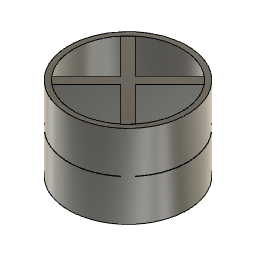
Moen Faucet Tool v1 (Autodesk Fusion 360 design; units mm, degrees)
Autodesk Fusion 360 part; units mm, degrees
note: some values were not read from the file. Set by a fixed rule: which sketch regions a step uses.
sketch "Tool" plane through (0, 0, 0) normal (0, 0, 1) x (1, 0, 0)
  circle A0 centre (0, 0) radius 10.415
  circle A1 centre (0, 0) radius 9.6
  line L0 (-10.415, 0.0013) -> (10.415, 0.0013) construction
  line L1 (0, 10.485) -> (0, -10.415) construction
  line L2 (-10.415, -0.7737) -> (10.415, -0.7737)
  line L3 (-10.415, 0.7763) -> (10.415, 0.7763)
  line L4 (-0.775, 10.485) -> (-0.775, -10.415)
  line L5 (0.775, 10.485) -> (0.775, -10.415)
  circle A2 centre (0, 0) radius 11.415
  dimension "d5" = 20.83
  dimension "d6" = 19.2
  dimension "d7" = 0.775
  dimension "d8" = -0.775
  dimension "d9" = 0.775
  dimension "d10" = -0.775
  dimension "d13" = 1
  constraint coincident A0.centre A1.centre
  constraint concentric A0 A1
  constraint coincident A0 L0.end
  constraint horizontal L0
  constraint coincident A0 L0.start
  constraint coincident A0 L1.end
  constraint perpendicular L0 L1
  measures "d5" diameter of A0
  measures "d6" diameter of A1
extrude "Extrude1" add sketch "Tool" against normal blind 8 contours A0 A1 L2 L3 | A0 A1 L4 L5 | A0 A1 L4 L5 | A0 A1 L2 L3 | A2
move_face "OffsetFaces1" offset -0.05 17 faces at (10.7291, 0.0008, 0) (1.7545, 10.2662, -5.3333) (9.5752, 0.6902, -5.3333) (8.0289, -6.6339, -5.3333) (9.8411, 0.7763, -2.6667) (9.8413, -0.7737, -2.6667) (0.775, 10.1136, -5.3333) (-0.603, 9.581, -5.3333) (-7.0069, 7.7056, -5.3333) (-10.1137, -0.7737, -2.6667) (-0.775, 10.1136, -2.6667) (0.775, -9.8412, -5.3333) (0.603, -9.581, -5.3333) (-1.2662, -10.3377, -5.3333) (-9.5904, -0.4296, -5.3333) (-0.775, -9.8412, -2.6667) (-10.1135, 0.7763, -2.6667)
sketch "Sketch2" plane through (0, 0, -0.05) normal (0, 0, 1) x (-1, 0, 0)
  arc A0 (-9.6228, 0.7237) -> (-9.6226, -0.7263) centre (0, 0) ccw
  line L0 (-9.6228, 0.7237) -> (-10.4399, 0.7237)
  arc A1 (-0.725, 10.4399) -> (-10.4399, 0.7237) centre (0, 0) ccw
  line L1 (-0.725, 10.4399) -> (-0.725, 9.6227)
  arc A2 (0.725, 9.6227) -> (-0.725, 9.6227) centre (0, 0) ccw
  line L2 (0.725, 9.6227) -> (0.725, 10.4399)
  arc A3 (10.4399, 0.7237) -> (0.725, 10.4399) centre (0, 0) ccw
  line L3 (10.4399, 0.7237) -> (9.6228, 0.7237)
  arc A4 (9.6226, -0.7263) -> (9.6228, 0.7237) centre (0, 0) ccw
  line L4 (9.6226, -0.7263) -> (10.4398, -0.7263)
  arc A5 (0.725, -10.4399) -> (10.4398, -0.7263) centre (0, 0) ccw
  line L5 (0.725, -10.4399) -> (0.725, -9.6227)
  arc A6 (-0.725, -9.6227) -> (0.725, -9.6227) centre (0, 0) ccw
  line L6 (-0.725, -9.6227) -> (-0.725, -10.4399)
  arc A7 (-10.4398, -0.7263) -> (-0.725, -10.4399) centre (0, 0) ccw
  line L7 (-10.4398, -0.7263) -> (-9.6226, -0.7263)
  circle A8 centre (0, 0) radius 11.415
  line L8 (0, 0) -> (8.0716, -8.0716) construction
  line L9 (0, 0) -> (11.415, 0) construction
  line L10 (0, 0) -> (8.0716, 8.0716) construction
  line L11 (0, 0) -> (11.415, 0) construction
  line L12 (0, 0) -> (-8.0716, -8.0716) construction
  line L13 (0, 0) -> (-8.0716, 8.0716) construction
  line L14 (0.7071, 0.7071) -> (8.7787, -7.3645)
  line L15 (0.7071, 0.7071) -> (-7.3645, 8.7787)
  line L16 (-0.7071, -0.7071) -> (-8.7787, 7.3645)
  line L17 (-0.7071, -0.7071) -> (7.3645, -8.7787)
  line L18 (0.7071, -0.7071) -> (8.7787, 7.3645)
  line L19 (0.7071, -0.7071) -> (-7.3645, -8.7787)
  line L20 (-0.7071, 0.7071) -> (7.3645, 8.7787)
  line L21 (-0.7071, 0.7071) -> (-8.7787, -7.3645)
  dimension "d17" = 45
  dimension "d18" = 45
  dimension "d19" = 90
  dimension "d20" = 1
  dimension "d21" = -1
  dimension "d22" = 1
  dimension "d23" = -1
  constraint horizontal L9
  constraint coincident A0.centre A1.centre
  constraint horizontal L11
  constraint coincident A8 L10.end
  constraint coincident A8 L12.end
  constraint perpendicular L8 L12
  constraint coincident A8 L13.end
  measures "d17" angle of L8 L9
  measures "d18" angle of L10 L11
  measures "d19" angle of L12 L13
extrude "Extrude2" add sketch "Sketch2" along normal blind 8 and the other way blind 2 contours A1 A8 L15 L16 | A1 L15 L16 L20 L21 | A7 L16 L17 L19 L21 | A7 A8 L19 L21 | L14 L15 L16 L17 L18 L19 L20 L21 | A3 L14 L15 L18 L20 | A5 L14 L17 L18 L19 | A3 A8 L18 L20 | A5 A8 L14 L17
extrude "Extrude3" add sketch "Tool" along normal blind 8
equation "outside_diamter = 20.83 mm"
equation "wall_thickness = 1.63 mm"
equation "tool_teeth_width = 1.55 mm"
equation "inside_diamter = outside_diamter - wall_thickness"
equation "d5 = outside_diamter"
equation "d6 = inside_diamter"
equation "d7 = tool_teeth_width / 2"
equation "d8 = -( tool_teeth_width / 2 )"
equation "d9 = tool_teeth_width / 2"
equation "d10 = -( tool_teeth_width / 2 )"
equation "tool_thickness = 1 mm"
equation "tool_depth = 8 mm"
equation "d13 = tool_thickness"
equation "d14 = -tool_depth"
